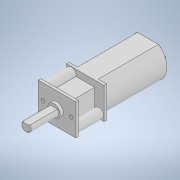
# Autodesk Inventor part: N30 gear motor
Saved by Autodesk Inventor 2020.2 (Build 242310000, 310)
## iProperties
Created: 2020-02-19
Part Number: N30 gear motor
Material: Generic
Document SubType Name: Modeling
Designer: mulve
Density: 1 g/cm^3
Appearance: Default
Author: mulve
Autodesk Inventor part; units mm, degrees
ref_plane "YZ Plane" through (0, 0, 0) normal (1, 0, 0) x (0, 1, 0)
ref_plane "XZ Plane" through (0, 0, 0) normal (0, 1, 0) x (-1, 0, 0)
sketch "Sketch1" plane through (0, 0, 0) normal (0, 0, 1) x (1, 0, 0)
  line L0 (0, 0) -> (12, 0)
  line L1 (12, 0) -> (12, 10)
  line L2 (12, 10) -> (0, 10)
  line L3 (0, 10) -> (0, 0)
  dimension "d0" = 10
  dimension "d1" = 12
  constraints: 8 end point, 2 parallel, 1 horizontal, 1 perpendicular
  measures "d0" distance of L2.end L0.start
  measures "d1" distance of L1.end L2.end
extrude "Extrusion1" add sketch "Sketch1" along normal blind 20
sketch "Sketch2" plane through (0, 0, 20) normal (0, 0, 1) x (1, 0, 0)
  line L0 (12, 0) -> (12, 10) projected
  line L1 (0, 0) -> (12, 0)
  line L2 (12, 0) -> (12, 10)
  line L3 (12, 10) -> (0, 10)
  line L4 (0, 10) -> (0, 0)
  constraints: 8 end point, 2 parallel, 1 horizontal, 1 perpendicular
extrude "Extrusion2" add sketch "Sketch2" along normal blind 9
sketch "Sketch3" plane through (0, 0, 29) normal (0, 0, 1) x (1, 0, 0)
  line L0 (12, 10) -> (0, 10) projected
  line L1 (0, 10) -> (0, 0) projected
  line L2 (12, 0) -> (12, 10) projected
  point P0 (1.5, 5)
  point P1 (10.5, 5)
  dimension "d6" = 5
  dimension "d7" = 5
  dimension "d8" = 9
  dimension "d9" = 1.5
  dimension "d10" = 1.5
  measures "d6" distance from line of L0 point (1.5, 5)
  measures "d7" distance from line of L0 point (10.5, 5)
  measures "d8" distance of point (10.5, 5) point (1.5, 5)
  measures "d9" distance from line of L1 point (1.5, 5)
  measures "d10" distance from line of L2 point (10.5, 5)
hole "Hole1" at (1.5, 5, 29) at (10.5, 5, 29) direction (0, 0, -1) diameter 1.221 depth 0.8 thread size "M1.6x0.35" class "6H" standard "ISO Metric profile"
ref_plane "Work Plane1" through (0, 0, 28.2) normal (0, 0, 1) x (1, 0, 0)
sketch "Sketch4" plane through (0, 0, 28.2) normal (0, 0, 1) x (1, 0, 0)
  line L0 (0, 10) -> (0, 0) projected
  line L1 (12, 0) -> (12, 10) projected
  line L2 (0, 0) -> (12, 0)
  line L3 (12, 0) -> (12, 10)
  line L4 (12, 10) -> (0, 10)
  line L5 (0, 10) -> (0, 0)
  line L6 (3, 2) -> (9, 2)
  line L7 (9, 2) -> (9, 8)
  line L8 (9, 8) -> (3, 8)
  line L9 (3, 8) -> (3, 2)
  circle A0 centre (10.5, 5) radius 0.6105 projected
  circle A1 centre (1.5, 5) radius 0.6105 projected
  point P0 (6, 5)
  dimension "d19" = 2
  dimension "d20" = 2
  dimension "d21" = 1.5
  dimension "d22" = 1.5
  constraints: 16 end point, 4 parallel, 2 horizontal, 2 perpendicular
  measures "d19" distance between parallel lines of L4 L8
  measures "d20" distance between parallel lines of L2 L6
  measures "d21" distance from line of A0.centre L7
  measures "d22" distance from line of A1.centre L9
extrude "Extrusion3" cut sketch "Sketch4" against normal blind 8.2 contours L4 L1 L2 L0 | A0 | A1
sketch "Sketch5" plane through (0, 0, 28.2) normal (0, 0, 1) x (1, 0, 0)
  line L0 (12, 10) -> (0, 10) projected
  line L1 (0, 10) -> (0, 0) projected
  line L2 (12, 0) -> (12, 10) projected
  line L3 (0, 0) -> (12, 0) projected
  circle A0 centre (1.6, 8.4) radius 1.5
  circle A1 centre (10.4, 1.6) radius 1.5
  dimension "d25" = 1.6
  dimension "d26" = 1.6
  dimension "d27" = 1.6
  dimension "d28" = 1.6
  dimension "d29" = 3
  constraints: 2 centre point, 2 coincident, 1 equal radius
  measures "d25" distance from line of L0 point (1.6, 8.4)
  measures "d26" distance from line of L1 point (1.6, 8.4)
  measures "d27" distance from line of L2 point (10.4, 1.6)
  measures "d28" distance from line of L3 point (10.4, 1.6)
  measures "d29" diameter of A0
extrude "Extrusion4" add sketch "Sketch5" against normal up to surface (8.2 mm away) contours A0 | A1
sketch "Sketch6" plane through (0, 0, 29) normal (0, 0, 1) x (1, 0, 0)
  line L0 (12, 10) -> (0, 10) projected
  line L1 (0, 0) -> (12, 0) projected
  line L2 (12, 0) -> (12, 10) projected
  line L3 (0, 10) -> (0, 0) projected
  circle A0 centre (6, 5) radius 2
  dimension "d32" = 5
  dimension "d33" = 5
  dimension "d34" = 6
  dimension "d35" = 6
  dimension "d36" = 4
  constraints: 1 centre point, 1 coincident
  measures "d32" distance from line of L0 point (6, 5)
  measures "d33" distance from line of L1 point (6, 5)
  measures "d34" distance from line of L2 point (6, 5)
  measures "d35" distance from line of L3 point (6, 5)
  measures "d36" diameter of A0
extrude "Extrusion5" add sketch "Sketch6" along normal blind 1 contours A0
sketch "Sketch7" plane through (6, 5, 30) normal (0, 0, 1) x (1, 0, 0)
  circle A0 centre (0, -0.0104) radius 1.5
  line L0 (-1.118, 0.9896) -> (1.118, 0.9896)
  point P0 (-6, -5)
  point P1 (0, -1.5104)
  dimension "d39" = 3
  dimension "d40" = 2.5
  constraints: 3 point on circle, 2 end point, 1 centre point, 1 horizontal
  measures "d39" diameter of A0
  measures "d40" distance from line of A0.start L0
extrude "Extrusion6" add sketch "Sketch7" along normal blind 9 contours A0 L0 picked at (0.0594, 0.1598)
chamfer "Chamfer1" distance 0.3 angle 45 1 edges at (6, 3.4896, 39)
sketch "Sketch8" plane through (0, 0, 0) normal (0, 0, -1) x (-1, 0, 0)
  line L0 (-12, 10) -> (0, 10) projected
  line L1 (-12, 0) -> (-12, 10) projected
  circle A0 centre (-6, 5) radius 6
  line L2 (-12, 10) -> (-12, 0) projected
  line L3 (0, 0) -> (-12, 0)
  line L4 (-12, 0) -> (-12, 10)
  line L5 (-12, 10) -> (0, 10)
  line L6 (0, 10) -> (0, 0)
  point P0 (0, 5)
  point P1 (0, 10)
  point P2 (-2.6834, 10)
  point P3 (-2.6834, 0)
  point P4 (-9.3166, 0)
  point P5 (-12, 5)
  point P6 (-9.3166, 10)
  dimension "d46" = 5
  dimension "d47" = 6
  constraints: 8 end point, 2 parallel, 1 centre point, 1 coincident, 1 horizontal, 1 perpendicular
  measures "d46" distance from line of L0 point (-6, 5)
  measures "d47" distance from line of L1 point (-6, 5)
extrude "Extrusion7" cut sketch "Sketch8" against normal blind 19.2 contours L0 A0 L1 | A0 L3 L1 | L0 L6 A0 | L6 L3 A0
sketch "Sketch9" plane through (0, 0, 0) normal (0, 0, -1) x (-1, 0, 0)
  arc A0 (-9.3166, 10) -> (-9.3166, 0) centre (-6, 5) ccw projected
  line L0 (-12, 5) -> (-12, 10) projected
  line L1 (0, 5) -> (0, 0) projected
  line L2 (-9.3, 4.25) -> (-9.6, 4.25)
  line L3 (-9.6, 4.25) -> (-9.6, 5.75)
  line L4 (-9.6, 5.75) -> (-9.3, 5.75)
  line L5 (-9.3, 5.75) -> (-9.3, 4.25)
  line L6 (-9.3, 4.25) -> (-9.6, 5.75) construction
  line L7 (-9.6, 4.25) -> (-9.3, 5.75) construction
  line L8 (-2.7, 4.25) -> (-2.4, 4.25)
  line L9 (-2.4, 4.25) -> (-2.4, 5.75)
  line L10 (-2.4, 5.75) -> (-2.7, 5.75)
  line L11 (-2.7, 5.75) -> (-2.7, 4.25)
  line L12 (-2.7, 4.25) -> (-2.4, 5.75) construction
  line L13 (-2.4, 4.25) -> (-2.7, 5.75) construction
  point P0 (-9.45, 5)
  point P1 (-2.55, 5)
  dimension "d50" = 6.9
  dimension "d51" = 0
  dimension "d52" = 0
  dimension "d53" = 2.55
  dimension "d54" = 2.55
  dimension "d55" = 1.5
  dimension "d56" = 0.3
  constraints: 24 end point, 4 midpoint, 4 parallel, 2 horizontal, 2 perpendicular, 1 collinear, 1 point on line
  measures "d50" distance of point (-9.45, 5) point (-2.55, 5)
  measures "d51" vertical distance of point (-9.45, 5) point (-2.55, 5)
  measures "d52" vertical distance of A0.centre point (-9.45, 5)
  measures "d53" distance from line of L0 point (-9.45, 5)
  measures "d54" distance from line of L1 point (-2.55, 5)
  measures "d55" distance of L2.end L3.end
  measures "d56" distance of L3.end L4.end
extrude "Extrusion8" add sketch "Sketch9" along normal blind 2
sketch "Sketch10" plane through (0, 0, 0) normal (0, 0, -1) x (-1, 0, 0)
  line L0 (-9.3166, 10) -> (-2.6834, 10) projected
  line L1 (-12, 0) -> (-12, 5) projected
  circle A0 centre (-6, 5) radius 2.5
  point P0 (0, 0)
  dimension "d59" = 5
  dimension "d60" = 6
  dimension "d61" = 5
  constraints: 1 centre point, 1 coincident
  measures "d59" distance from line of L0 point (-6, 5)
  measures "d60" distance from line of L1 point (-6, 5)
  measures "d61" diameter of A0
extrude "Extrusion9" add sketch "Sketch10" along normal blind 1.1
equation "\"d7\" = d6"
equation "\"d9\" = d10"
equation "\"d20\" = d19"
equation "\"d22\" = d21"
equation "\"d26\" = d25"
equation "\"d27\" = d26"
equation "\"d28\" = d27"
equation "\"d32\" = d33"
equation "\"d34\" = d35"
equation "\"d53\" = d54"
body "Solid1"
